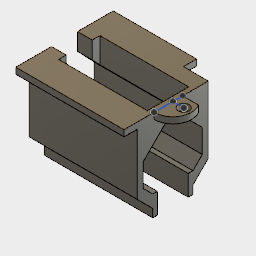
Pelvis (x4) (Autodesk Fusion 360 design; units mm, degrees)
Autodesk Fusion 360 part; units mm, degrees
sketch "Sketch1" plane through (0, 0, 0) normal (0, 1, 0) x (1, 0, 0)
  line L0 (0, 0) -> (0, 11.5)
  line L1 (0, 0) -> (0, -8.3) construction
  line L2 (0, -8.3) -> (0, -19.8)
  line L3 (0, -19.8) -> (34.75, -19.8)
  line L4 (34.75, -19.8) -> (34.75, -10.025)
  line L5 (0, 11.5) -> (26.75, 11.5)
  line L6 (26.75, 11.5) -> (26.75, 7.25)
  line L7 (26.75, 7.25) -> (34.75, 7.25)
  line L8 (34.75, 7.25) -> (34.75, 1.85)
  line L9 (0, 0) -> (4.75, 0)
  line L10 (0, -8.3) -> (4.75, -8.3)
  line L11 (4.75, 0) -> (4.75, 2.475)
  line L12 (4.75, 2.475) -> (33.25, 2.475)
  line L13 (4.75, -8.3) -> (4.75, -10.775)
  line L14 (4.75, -10.775) -> (33.25, -10.775)
  line L15 (33.25, -10.775) -> (33.25, 2.475)
  line L16 (33.25, -4.15) -> (34.75, -4.15)
  arc A0 (34.75, -10.15) -> (34.75, 1.85) centre (34.75, -4.15) ccw
  line L17 (33.25, -4.15) -> (38.25, -4.15)
  circle A1 centre (38.25, -4.15) radius 1.75
  dimension "d1" = 11.5
  dimension "d2" = 8.3
  dimension "d3" = 11.5
  dimension "d4" = 34.75
  dimension "d5" = 9.775
  dimension "d6" = 26.75
  dimension "d7" = 4.25
  dimension "d8" = 8
  dimension "d10" = 4.75
  dimension "d11" = 4.75
  dimension "d12" = 2.475
  dimension "d13" = 28.5
  dimension "d14" = 2.475
  dimension "d15" = 28.5
  dimension "d16" = 12
  dimension "d17" = 5
  dimension "d18" = 3.5
  measures "d1" distance of L0.start L0.end
  measures "d2" distance of L0.start L1.end
  measures "d3" distance of L1.end L2.end
  measures "d4" distance of L2.end L3.end
  measures "d5" distance of L3.end L4.end
  measures "d6" distance of L0.end L5.end
  measures "d7" distance of L5.end L6.end
  measures "d8" distance of L6.end L7.end
  measures "d10" distance of L0.start L9.end
  measures "d11" distance of L1.end L10.end
  measures "d12" distance of L9.end L11.end
  measures "d13" distance of L11.end L12.end
  measures "d14" distance of L10.end L13.end
  measures "d15" distance of L13.end L14.end
  measures "d16" diameter of A0
  measures "d17" distance of L16.start L17.end
  measures "d18" diameter of A1
extrude "Extrude1" add sketch "Sketch1" against normal blind 2
sketch "Sketch2" plane through (0, 0, 0) normal (-1, 0, 0) x (0, 0, 1)
  line L0 (0, 0) -> (-11.5, 0)
  line L1 (-11.5, 0) -> (-11.5, -2)
  line L2 (-11.5, -2) -> (0, -2)
  line L3 (0, -2) -> (0, 0)
  line L4 (0, -2) -> (0, -5.535)
  line L5 (8.3, -2) -> (8.3, -5.535)
  line L6 (0, -2) -> (-7.25, -2) construction
  line L7 (8.3, -2) -> (15.55, -2) construction
  line L8 (-7.25, -2) -> (-7.25, -21.5)
  line L9 (15.55, -2) -> (15.55, -21.5)
  line L10 (-7.25, -21.5) -> (-2.3003, -26.4497)
  line L11 (-7.25, -21.5) -> (-0.25, -21.5) construction
  line L12 (15.55, -21.5) -> (10.6003, -26.4497)
  line L13 (15.55, -21.5) -> (22.55, -21.5) construction
  line L14 (-2.3003, -26.4497) -> (-2.3003, -29.5997)
  line L15 (10.6003, -26.4497) -> (10.6003, -29.5997)
  line L16 (-2.3003, -29.5997) -> (10.6003, -29.5997)
  line L17 (-2.3003, -29.5997) -> (-2.3003, -22.4497) construction
  line L18 (10.6003, -29.5997) -> (10.6003, -22.4497) construction
  line L19 (10.6003, -22.4497) -> (-2.3003, -22.4497)
  line L20 (-2.3003, -22.4497) -> (-5.3055, -19.4445)
  line L21 (-2.3003, -22.4497) -> (1.9497, -22.4497) construction
  line L22 (10.6003, -22.4497) -> (13.6055, -19.4445)
  line L23 (10.6003, -22.4497) -> (14.8503, -22.4497) construction
  line L24 (-5.3055, -19.4445) -> (-5.3055, -11.0945)
  line L25 (13.6055, -19.4445) -> (13.6055, -11.0945)
  line L26 (-5.3055, -11.0945) -> (0, -5.535)
  line L27 (13.6055, -11.0945) -> (8.3, -5.535)
  line L28 (-7.25, -2) -> (0, -2)
  line L29 (8.3, -2) -> (15.55, -2)
  point P0 (8.3, -2)
  dimension "d24" = 3.535
  dimension "d25" = 3.535
  dimension "d26" = 7.25
  dimension "d27" = 7.25
  dimension "d28" = 19.5
  dimension "d29" = 19.5
  dimension "d30" = 45
  dimension "d31" = 7
  dimension "d32" = 135
  dimension "d33" = 7
  dimension "d34" = 3.15
  dimension "d35" = 3.15
  dimension "d36" = 7.15
  dimension "d37" = 7.15
  dimension "d38" = 135
  dimension "d39" = 4.25
  dimension "d40" = 45
  dimension "d41" = 4.25
  dimension "d42" = 8.35
  dimension "d43" = 8.35
  measures "d24" distance of L2.end L4.end
  measures "d25" distance of P0 L5.end
  measures "d26" distance of L2.end L6.end
  measures "d27" distance of P0 L7.end
  measures "d28" distance of L6.end L8.end
  measures "d29" distance of L7.end L9.end
  measures "d30" angle of L10 L11
  measures "d31" distance of L8.end L10.end
  measures "d32" angle of L12 L13
  measures "d33" distance of L9.end L12.end
  measures "d34" distance of L10.end L14.end
  measures "d35" distance of L12.end L15.end
  measures "d36" distance of L14.end L17.end
  measures "d37" distance of L15.end L18.end
  measures "d38" angle of L20 L21
  measures "d39" distance of L17.end L20.end
  measures "d40" angle of L22 L23
  measures "d41" distance of L18.end L22.end
  measures "d42" distance of L20.end L24.end
  measures "d43" distance of L22.end L25.end
extrude "Extrude2" add sketch "Sketch2" against normal blind 34.75 contours L2 L4 L5 L8 L9 L10 L12 L14 L15 L16 L19 L20 L22 L24 L25 L26 L27 L28 L29
extrude "Extrude3" cut 2 faces at (14.25, -2, -1.65) (23.75, -2, 9.125) along direction (0, -1, 0) blind 10
sketch "Sketch3" plane through (0, 0, 0) normal (0, 1, 0) x (-1, 0, 0)
  circle A0 centre (-38.25, 4.15) radius 1.75
  line L0 (0, 8.3) -> (0, 19.8)
  line L1 (0, 19.8) -> (-34.75, 19.8)
  line L2 (-34.75, 19.8) -> (-34.75, 10.15)
  arc A1 (-34.75, 10.15) -> (-34.75, -1.85) centre (-34.75, 4.15) ccw
  line L3 (-34.75, -1.85) -> (-34.75, -7.25)
  line L4 (-34.75, -7.25) -> (-26.75, -7.25)
  line L5 (-26.75, -7.25) -> (-26.75, -11.5)
  line L6 (-26.75, -11.5) -> (0, -11.5)
  line L7 (0, -11.5) -> (0, 0)
  line L8 (0, 0) -> (-4.75, 0)
  line L9 (-4.75, 0) -> (-4.75, -2.475)
  line L10 (-4.75, -2.475) -> (-33.25, -2.475)
  line L11 (-33.25, -2.475) -> (-33.25, 10.775)
  line L12 (-33.25, 10.775) -> (-4.75, 10.775)
  line L13 (-4.75, 10.775) -> (-4.75, 8.3)
  line L14 (-4.75, 8.3) -> (0, 8.3)
  line L15 (-34.75, -1.85) -> (-34.75, 1.025)
  line L16 (-34.75, 1.025) -> (-41.4539, 1.025)
  dimension "d48" = 2.875
  measures "d48" distance of A1.end L15.end
extrude "Extrude4" cut sketch "Sketch3" against normal blind 13 contours A1 L15 L16
sketch "Sketch4" plane through (34.75, 0, 0) normal (1, 0, 0) x (0, 0, -1)
  line L0 (0, -5.535) -> (5.3055, -11.0945)
  line L1 (5.3055, -11.0945) -> (5.3055, -19.4445)
  line L2 (5.3055, -19.4445) -> (2.3003, -22.4497)
  line L3 (2.3003, -22.4497) -> (-10.6003, -22.4497)
  line L4 (-10.6003, -22.4497) -> (-13.6055, -19.4445)
  line L5 (-13.6055, -19.4445) -> (-13.6055, -11.0945)
  line L6 (-13.6055, -11.0945) -> (-8.3, -5.535)
  line L7 (-8.3, -5.535) -> (-8.3, -2)
  line L8 (-8.3, -2) -> (-10.15, -2)
  line L9 (-10.15, -2) -> (-10.15, 0)
  line L10 (-10.15, 0) -> (-19.8, 0)
  line L11 (-19.8, 0) -> (-19.8, -2)
  line L12 (-19.8, -2) -> (-15.55, -2)
  line L13 (-15.55, -2) -> (-15.55, -21.5)
  line L14 (-15.55, -21.5) -> (-10.6003, -26.4497)
  line L15 (-10.6003, -26.4497) -> (-10.6003, -29.5997)
  line L16 (-10.6003, -29.5997) -> (2.3003, -29.5997)
  line L17 (2.3003, -29.5997) -> (2.3003, -26.4497)
  line L18 (2.3003, -26.4497) -> (7.25, -21.5)
  line L19 (7.25, -21.5) -> (7.25, 0)
  line L20 (7.25, 0) -> (-1.025, 0)
  line L21 (-1.025, 0) -> (-1.025, -2)
  line L22 (-1.025, -2) -> (0, -2)
  line L23 (0, -2) -> (0, -5.535)
  line L24 (-3.535, -2) -> (-3.6055, -1.9295)
  line L25 (0, -5.535) -> (10, -5.535) construction
  line L26 (-4.765, -2) -> (-4.6945, -1.9295)
  line L27 (-8.3, -5.535) -> (1.7, -5.535) construction
  line L28 (-16, -15) -> (-15.5, -15)
  line L29 (-13.6055, -11.0945) -> (-13.6055, -11.9295)
  line L30 (-13.6055, -11.9295) -> (6.3945, -11.9295) construction
  line L31 (5.3055, -11.0945) -> (5.3055, -11.9295)
  line L32 (5.3055, -11.9295) -> (25.3055, -11.9295) construction
  line L33 (-8.3, -5.535) -> (-8.3, -2)
  line L34 (-8.3, -2) -> (0, -2)
  line L35 (0, -2) -> (0, -5.535)
  line L36 (0, -5.535) -> (5.3055, -11.0945)
  line L37 (-13.6055, -11.9295) -> (-4.15, -2.4741)
  line L38 (-3.6759, -2) -> (-3.6055, -1.9295)
  line L39 (5.3055, -11.9295) -> (-4.15, -2.4741)
  line L40 (-4.6241, -2) -> (-4.6945, -1.9295)
  dimension "d51" = 135
  dimension "d53" = 45
  dimension "d55" = 0.835
  dimension "d56" = 45
  dimension "d58" = 0.835
  dimension "d59" = 135
  measures "d51" angle of L24 L25
  measures "d53" angle of L26 L27
  measures "d55" distance of L5.end L29.end
  measures "d56" angle of L30 L37
  measures "d58" distance of L0.end L31.end
  measures "d59" angle of L32 L39
extrude "Extrude5" add sketch "Sketch4" against normal blind 1.5 contours L0 L1 L5 L6 L7 L22 L23 L29 L31 L33 L34 L35 L36 L37 L39
sketch "Sketch5" plane through (0, -29.5997, 0) normal (0, -1, 0) x (1, 0, 0)
  line L0 (0, 10.6003) -> (0, -2.3003)
  line L1 (0, -2.3003) -> (34.75, -2.3003)
  line L2 (34.75, -2.3003) -> (34.75, 10.6003)
  line L3 (34.75, 10.6003) -> (0, 10.6003)
  line L4 (0, 4.15) -> (12.25, 4.15)
  circle A0 centre (12.25, 4.15) radius 3.5
  dimension "d63" = 12.25
  dimension "d65" = 7
  measures "d63" distance of L4.start L4.end
  measures "d65" diameter of A0
extrude "Extrude6" cut sketch "Sketch5" against normal blind 13 contours A0
sketch "Sketch6" plane through (34.75, 0, 0) normal (1, 0, 0) x (0, 0, -1)
  line L0 (-1.025, -2) -> (-10.15, -2)
  line L1 (-10.15, -2) -> (-10.15, 0)
  line L2 (-10.15, 0) -> (-19.8, 0)
  line L3 (-19.8, 0) -> (-19.8, -2)
  line L4 (-19.8, -2) -> (-15.55, -2)
  line L5 (-15.55, -2) -> (-15.55, -21.5)
  line L6 (-15.55, -21.5) -> (-10.6003, -26.4497)
  line L7 (-10.6003, -26.4497) -> (-10.6003, -29.5997)
  line L8 (-10.6003, -29.5997) -> (2.3003, -29.5997)
  line L9 (2.3003, -29.5997) -> (2.3003, -26.4497)
  line L10 (2.3003, -26.4497) -> (7.25, -21.5)
  line L11 (7.25, -21.5) -> (7.25, 0)
  line L12 (7.25, 0) -> (-1.025, 0)
  line L13 (-1.025, 0) -> (-1.025, -2)
  line L14 (-13.6055, -11.9295) -> (-4.15, -2.4741)
  line L15 (-4.15, -2.4741) -> (5.3055, -11.9295)
  line L16 (5.3055, -11.9295) -> (5.3055, -19.4445)
  line L17 (5.3055, -19.4445) -> (2.3003, -22.4497)
  line L18 (2.3003, -22.4497) -> (-10.6003, -22.4497)
  line L19 (-10.6003, -22.4497) -> (-13.6055, -19.4445)
  line L20 (-13.6055, -19.4445) -> (-13.6055, -11.9295)
  line L21 (2.3003, -29.5997) -> (0.8003, -29.5997)
  line L22 (-10.6003, -29.5997) -> (-9.1003, -29.5997)
  line L23 (-9.1003, -29.5997) -> (-9.1003, -22.4494)
  line L24 (0.8003, -29.5997) -> (0.8003, -22.4497)
  dimension "d69" = 1.5
  dimension "d70" = 1.5
  dimension "d71" = 7.15
  measures "d69" distance of L8.end L21.end
  measures "d70" distance of L7.end L22.end
  measures "d71" distance of L21.end L24.end
extrude "Extrude7" cut sketch "Sketch6" against normal blind 16 contours L8 L18 L23 L24
sketch "Sketch7" plane through (0, 0, 0) normal (-1, 0, 0) x (0, 0, 1)
  line L0 (0, 0) -> (-11.5, 0)
  line L1 (-11.5, 0) -> (-11.5, -2)
  line L2 (-11.5, -2) -> (-7.25, -2)
  line L3 (-7.25, -2) -> (-7.25, -21.5)
  line L4 (-7.25, -21.5) -> (-2.3003, -26.4497)
  line L5 (-2.3003, -26.4497) -> (-2.3003, -29.5997)
  line L6 (-2.3003, -29.5997) -> (10.6003, -29.5997)
  line L7 (10.6003, -29.5997) -> (10.6003, -26.4497)
  line L8 (10.6003, -26.4497) -> (15.55, -21.5)
  line L9 (15.55, -21.5) -> (15.55, -2)
  line L10 (15.55, -2) -> (19.8, -2)
  line L11 (19.8, -2) -> (19.8, 0)
  line L12 (19.8, 0) -> (8.3, 0)
  line L13 (8.3, 0) -> (8.3, -5.535)
  line L14 (8.3, -5.535) -> (13.6055, -11.0945)
  line L15 (13.6055, -11.0945) -> (13.6055, -19.4445)
  line L16 (13.6055, -19.4445) -> (10.6003, -22.4497)
  line L17 (10.6003, -22.4497) -> (-2.3003, -22.4497)
  line L18 (-2.3003, -22.4497) -> (-5.3055, -19.4445)
  line L19 (-5.3055, -19.4445) -> (-5.3055, -11.0945)
  line L20 (-5.3055, -11.0945) -> (0, -5.535)
  line L21 (0, -5.535) -> (0, 0)
  line L22 (10.6003, -29.5997) -> (9.1003, -29.5997)
  line L23 (-2.3003, -29.5997) -> (-0.8003, -29.5997)
  line L24 (-0.8003, -29.5997) -> (-0.8003, -22.4497)
  line L25 (9.1003, -29.5997) -> (9.1003, -22.4497)
  point P0 (-0.8003, -22.4497)
  point P1 (9.1003, -22.4497)
  dimension "d74" = 1.5
  dimension "d75" = 1.5
  measures "d74" distance of L6.end L22.end
  measures "d75" distance of L5.end L23.end
extrude "Extrude8" cut sketch "Sketch7" against normal blind 4.75 contours L6 L17 L24 L25
extrude "Extrude9" cut 1 faces at (6.0833, -29.5997, 4.15) along direction (0, 1, 0) blind 0.5
sketch "Sketch8" plane through (0, 0, 0) normal (0, 1, 0) x (-1, 0, 0)
  line L0 (-39.872, 1.025) -> (-34.75, 1.025)
  line L1 (-34.75, 1.025) -> (-34.75, -7.25)
  line L2 (-34.75, -7.25) -> (-26.75, -7.25)
  line L3 (-26.75, -7.25) -> (-26.75, -11.5)
  line L4 (-26.75, -11.5) -> (0, -11.5)
  line L5 (0, -11.5) -> (0, 0)
  line L6 (0, 0) -> (-4.75, 0)
  line L7 (-4.75, 0) -> (-4.75, -2.475)
  line L8 (-4.75, -2.475) -> (-33.25, -2.475)
  line L9 (-33.25, -2.475) -> (-33.25, 10.775)
  line L10 (-33.25, 10.775) -> (-4.75, 10.775)
  line L11 (-4.75, 10.775) -> (-4.75, 8.3)
  line L12 (-4.75, 8.3) -> (0, 8.3)
  line L13 (0, 8.3) -> (0, 19.8)
  line L14 (0, 19.8) -> (-34.75, 19.8)
  line L15 (-34.75, 19.8) -> (-34.75, 10.15)
  arc A0 (-34.75, 10.15) -> (-39.872, 1.025) centre (-34.75, 4.15) ccw
  circle A1 centre (-38.25, 4.15) radius 1.75
  line L16 (-34.75, 10.15) -> (-34.75, 1.025)
  line L17 (-34.75, 4.15) -> (-38.25, 4.15)
equation "d17 = HolePosX"
equation "d18 = HoleSize"
equation "HolePosX = 5 mm"
equation "HoleSize = 3.5 mm"
equation "d21 = -TopThickness"
equation "TopThickness = 2 mm"
equation "d63 = JointPosX"
equation "JointPosX = 12.25 mm"
equation "d65 = HoleBall"
equation "HoleBall = 7 mm"
